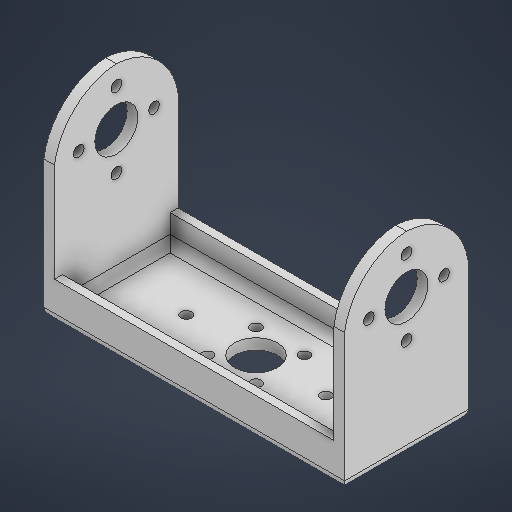
# Autodesk Inventor part: ShotFrame
Saved by Autodesk Inventor 2027 (Build 310192060, 192F)
## iProperties
Created: 2026-09-09
Part Number: ShotFrame
Material: Genérico
Document SubType Name: Modeling
Designer: paulo
Density: 1 g/cm^3
Appearance: Padrão
Author: paulo
Autodesk Inventor part; units mm, degrees
ref_plane "YZ Plane" through (0, 0, 0) normal (1, 0, 0) x (0, 1, 0)
ref_plane "XZ Plane" through (0, 0, 0) normal (0, 1, 0) x (-1, 0, 0)
ref_plane "XY Plane" through (0, 0, 0) normal (0, 0, 1) x (1, 0, 0)
sketch "Esboço1" plane through (0, 0, 0) normal (0, 1, 0) x (-1, 0, 0)
  line L0 (-25.9999, 11.4129) -> (25.9999, -11.4129) construction
  line L1 (28, 11.5) -> (-28, -11.5) construction
  circle A0 centre (0, 0) radius 4
  line L2 (26, 10) -> (-26, 10)
  line L3 (-26, 10) -> (-26, -10)
  line L4 (-26, -10) -> (26, -10)
  line L5 (26, -10) -> (26, 10)
  line L6 (26, 10) -> (-26, -10) construction
  line L7 (-26, 10) -> (26, -10) construction
  line L8 (13, 0) -> (-13, 0)
  circle A1 centre (-13, 0) radius 1
  circle A2 centre (13, 0) radius 1
  line L9 (4.5, 4.5) -> (-4.5, 4.5)
  line L10 (4.5, -4.5) -> (4.5, 4.5)
  line L11 (4.5, 4.5) -> (-4.5, -4.5) construction
  line L12 (-4.5, 4.5) -> (4.5, -4.5) construction
  circle A3 centre (4.5, 4.5) radius 1
  circle A4 centre (4.5, -4.5) radius 1
  circle A5 centre (-4.5, 4.5) radius 1
  circle A6 centre (-4.5, -4.5) radius 1
  line L13 (28, 11.5) -> (-28, 11.5)
  line L14 (-28, 11.5) -> (-28, -11.5)
  line L15 (-28, -11.5) -> (28, -11.5)
  line L16 (28, -11.5) -> (28, 11.5)
  line L17 (28, 11.5) -> (-28, -11.5) construction
  line L18 (-28, 11.5) -> (28, -11.5) construction
  line L19 (26, -10) -> (26, -11.5)
  line L20 (26, 10) -> (26, 11.5)
  line L21 (-26, 10) -> (-26, 11.5)
  line L22 (-26, -10) -> (-26, -11.5)
  dimension "d0" = 54
  dimension "d1" = 23
  dimension "d2" = 8
  dimension "d3" = 52
  dimension "d4" = 20
  dimension "d5" = 26
  dimension "d6" = 2
  dimension "d7" = 2
  dimension "d8" = 9
  dimension "d9" = 9
  dimension "d10" = 2
  dimension "d13" = 9
  dimension "d16" = 9
  dimension "d19" = 56
  dimension "d20" = 23
  constraints: 46 end point, 9 midpoint, 7 centre point, 5 horizontal, 5 perpendicular, 5 point on line, 4 coincident, 4 parallel, 1 vertical, 6 other
  measures "d0" distance of L0.end L1.end
  measures "d1" distance of L1.start L0.end
  measures "d2" diameter of A0
  measures "d3" distance of L4.end L3.end
  measures "d4" distance of L3.end L2.end
  measures "d5" distance of L8.start L8.end
  measures "d6" diameter of A1
  measures "d7" diameter of A2
  measures "d8" distance of L10.start L11.end
  measures "d9" distance of L11.end L9.end
  measures "d10" diameter of A3
  measures "d13" distance of A3.centre A4.centre
  measures "d16" distance of A3.centre A5.centre
  measures "d19" distance of L15.end L1.end
  measures "d20" distance of L1.end L13.end
extrude "Extrusão1" add sketch "Esboço1" along normal blind 34 and the other way blind 2 contours L20 L13 L16 L15 L19 L5 | L3 L22 L15 L14 L13 L21
extrude "Extrusão2" add sketch "Esboço1" along normal blind 5 and the other way blind 2 contours L2 L21 L13 L20 | L19 L15 L22 L4
extrude "Extrusão3" add sketch "Esboço1" against normal blind 2 contours L5 L4 L3 L2
sketch "Esboço3" plane through (-28, -2, -11.5) normal (-1, 0, 0) x (0, 0, 1)
  line L0 (11.5, 2) -> (11.5, 25.4)
  circle A0 centre (11.5, 25.4) radius 4
  line L1 (11.5, 25.4) -> (11.5, 18.4)
  circle A1 centre (11.5, 18.4) radius 1
  circle A2 centre (18.5, 25.4) radius 1
  circle A3 centre (11.5, 32.4) radius 1
  circle A4 centre (4.5, 25.4) radius 1
  line L2 (11.5, 2) -> (-22.5, 2)
  line L3 (7.5, 2) -> (15.5, 2) projected
  line L4 (11.5, 2) -> (11.5, 36)
  line L5 (-7.4457, 25.4) -> (30.4457, 25.4)
  line L6 (0, 36) -> (0, 7) projected
  arc A5 (11.5, 36) -> (0, 25.4) centre (12.2417, 23.6571) ccw
  arc A6 (23, 25.4) -> (11.5, 36) centre (10.7583, 23.6571) ccw
  line L7 (0, 0) -> (0, 36) projected
  line L8 (0, 25.4) -> (0, 36)
  line L9 (0, 36) -> (23, 36)
  line L10 (23, 36) -> (23, 25.4)
  point P0 (-22.5, 2)
  point P1 (11.5, 36)
  point P2 (11.5, 36)
  dimension "d27" = 23.4
  dimension "d28" = 8
  dimension "d29" = 7
  dimension "d30" = 2
  dimension "d33" = 360
  dimension "d39" = 34
  dimension "d40" = 34
  constraints: 14 end point, 7 centre point, 4 point on circle, 3 point on line, 2 coincident, 2 horizontal, 2 perpendicular, 2 vertical, 1 collinear, 1 midpoint, 12 other
  measures "d27" distance of L0.start L0.end
  measures "d28" diameter of A0
  measures "d29" distance of L1.start L1.end
  measures "d30" diameter of A1
  measures "d39" distance of L0.start point (-22.5, 2)
  measures "d40" distance of L0.start L4.end
extrude "Extrusão4" cut sketch "Esboço3" along normal blind 5.75 and the other way blind 76 contours A1 L0 | L0 A1 | A0 L5 L0 | L0 L5 A0 | L5 A0 L4 | L4 A0 L5 | L5 A4 | A4 L5 | L5 A2 | A2 L5 | L4 A3 | A3 L4
extrude "Extrusão5" cut sketch "Esboço3" along normal blind 5.75 and the other way blind 76 contours L6 L9 A5 | L9 L10 A6
fillet "Arredondamento2" radius 1.5 8 edges at (0, 0, 10) (-26, 0, 0) (0, 0, -10) (26, 0, 0) (0, -2, 11.5) (-28, -2, 0) (0, -2, -11.5) (28, -2, 0)
